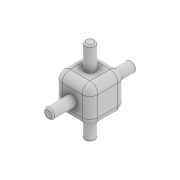
# Autodesk Inventor part: Ball
Saved by Autodesk Inventor 2020 (Build 240168000, 168)
## iProperties
Created: 2021-06-28
Part Number: Ball
Material: Generic
Document SubType Name: Modeling
Designer: Coy
Density: 1 g/cm^3
Appearance: Default
Author: Coy
Autodesk Inventor part; units mm, degrees
ref_plane "YZ Plane" through (0, 0, 0) normal (1, 0, 0) x (0, 1, 0)
ref_plane "XZ Plane" through (0, 0, 0) normal (0, 1, 0) x (-1, 0, 0)
ref_plane "XY Plane" through (0, 0, 0) normal (0, 0, 1) x (1, 0, 0)
sketch "Sketch1" plane through (0, 0, 0) normal (0, 0, 1) x (1, 0, 0)
  line L0 (0, 0) -> (-4.5, 0)
  line L1 (-4.5, 0) -> (-4.5, 4.5)
  line L2 (-4.5, 4.5) -> (0, 4.5)
  line L3 (0, 4.5) -> (0, 0)
  dimension "d0" = 4.5
  dimension "d1" = 4.5
  constraints: 8 end point, 2 parallel, 1 horizontal, 1 perpendicular
  measures "d0" distance of L1.end L2.end
  measures "d1" distance of L0.end L1.end
extrude "Extrusion1" add sketch "Sketch1" along normal blind 4.5
sketch "Sketch2" plane through (0, 0, 4.5) normal (0, 0, 1) x (1, 0, 0)
  line L0 (0, 4.5) -> (-4.5, 4.5) construction
  line L1 (-2.25, 4.5) -> (-2.25, 0) construction
  line L2 (-4.5, 0) -> (0, 0) construction
  circle A0 centre (-2.25, 2.25) radius 0.625
  dimension "d4" = 1.25
  constraints: 3 midpoint, 2 end point, 1 centre point
  measures "d4" diameter of A0
extrude "Extrusion2" add sketch "Sketch2" along normal blind 3
sketch "Sketch3" plane through (0, 0, 0) normal (0, 0, -1) x (-1, 0, 0)
  circle A0 centre (2.25, 2.25) radius 0.625 projected
  point P0 (0, 0)
extrude "Extrusion3" add sketch "Sketch3" along normal blind 3
sketch "Sketch4" plane through (-4.5, 4.5, 0) normal (0, 1, 0) x (1, 0, 0)
  line L0 (0, 0) -> (0, -4.5) construction
  line L1 (0, -2.25) -> (4.5, -2.25) construction
  line L2 (4.5, 0) -> (4.5, -4.5) construction
  circle A0 centre (2.25, -2.25) radius 0.625
  constraints: 3 midpoint, 2 end point, 1 centre point
extrude "Extrusion4" add sketch "Sketch4" along normal blind 3
sketch "Sketch5" plane through (-4.5, 0, 0) normal (0, -1, 0) x (1, 0, 0)
  circle A0 centre (2.25, 2.25) radius 0.625 projected
  point P0 (4.5, 0)
extrude "Extrusion5" add sketch "Sketch5" along normal blind 3
fillet "Fillet1" radius 1 12 edges at (-2.25, 4.5, 4.5) (-2.25, 0, 4.5) (-2.25, 0, 0) (-2.25, 4.5, 0) (0, 4.5, 2.25) (-4.5, 4.5, 2.25) (-4.5, 0, 2.25) (0, 0, 2.25) (0, 2.25, 0) (0, 2.25, 4.5) (-4.5, 2.25, 0) (-4.5, 2.25, 4.5)
fillet "Fillet2" radius 0.2 4 edges at (-2.875, 7.5, 2.25) (-2.875, 2.25, 7.5) (-1.625, 2.25, -3) (-2.875, -3, 2.25)
ref_plane "Work Plane1" through (-2.25, 1, 1) normal (-1, 0, 0) x (0, 0, 1)
sketch "Sketch8" plane through (-2.25, 1, 1) normal (-1, 0, 0) x (0, 0, 1)
  line L0 (-4, 0.825) -> (-4, 1.675) construction
  line L1 (-4, 1.25) -> (6.5, 1.25)
  line L2 (6.5, 1.675) -> (6.5, 0.825) construction
  arc A0 (1.75, 1.25) -> (0.75, 1.25) centre (1.25, 1.25) ccw
  point P0 (-1, -1)
  dimension "d19" = 1
  constraints: 3 midpoint, 2 end point, 2 point on circle, 2 point on line, 1 centre point
  measures "d19" diameter of A0
revolve "Revolution1" cut sketch "Sketch8" angle 360 about axis through (-2.25, 2.25, -3) along (0, 0, 1)
sketch "Sketch9" plane through (-4.5, 1, 1) normal (-1, 0, 0) x (0, 0, 1)
  line L0 (-1, 2.5) -> (0, 2.5) construction
  line L1 (-1, 2.5) -> (-1, 0) construction
  line L2 (-1, 2.5) -> (-1, 0) construction
  line L3 (-1, 1.25) -> (3.5, 1.25) construction
  line L4 (3.5, 2.5) -> (3.5, 0) construction
  circle A0 centre (1.25, 1.25) radius 0.5
  point P0 (-1, -1)
  constraints: 4 end point, 3 midpoint, 1 centre point, 1 vertical
extrude "Extrusion7" cut sketch "Sketch9" against normal up to next
body "Solid1"
